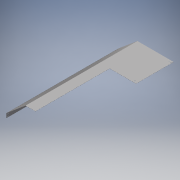
# Autodesk Inventor part: MC Part2
Saved by Autodesk Inventor 2016 (Build 200138000, 138)
## iProperties
Created: 2017-10-17
Part Number: MC Part2
Material: Steel, Mild
Document SubType Name: Sheet Metal
Designer: m207653
Density: 7.85 g/cm^3
Sheet Metal Rule: ms steel
Appearance: Semi-Polished
Flat Pattern Width: 99.3305 cm
Flat Pattern Length: 169.5 cm
Flat Pattern Area: 16836.5 cm^2
Sheet Metal Width: 993.305 mm
Sheet Metal Length: 1695.000 mm
Sheet Metal Area: 1683652.545 mm^2
Author: m207653
Autodesk Inventor part; units mm, degrees
ref_plane "YZ Plane" through (0, 0, 0) normal (1, 0, 0) x (0, 1, 0)
ref_plane "XZ Plane" through (0, 0, 0) normal (0, 1, 0) x (-1, 0, 0)
ref_plane "XY Plane" through (0, 0, 0) normal (0, 0, 1) x (1, 0, 0)
sketch "Sketch1" plane through (0, 0, 0) normal (0, 0, 1) x (1, 0, 0)
  line L0 (0, 0) -> (150, 0)
  line L1 (0, 0) -> (0, 1695)
  line L2 (0, 1695) -> (550, 1695)
  line L3 (550, 1695) -> (550, 1125)
  line L4 (550, 1125) -> (150, 1125)
  line L5 (150, 1125) -> (150, 0)
  dimension "d0" = 150
  dimension "d1" = 1695
  dimension "d2" = 550
  dimension "d3" = 570
  measures "d0" distance of L0.start L0.end
  measures "d1" distance of L0.start L1.end
  measures "d2" distance of L1.end L2.end
  measures "d3" distance of L2.end L3.end
extrude "Plate1" add sketch "Sketch1" along normal blind 1.6
sketch "Sketch2" plane through (1.0285, 0, 0.3743) normal (-0.6427876, 0, 0.7660444) x (0, -1, 0)
  line L0 (-1695, 0) -> (0, 0)
  line L1 (0, 0) -> (0, 380)
  line L2 (0, 380) -> (-1695, 380)
  line L3 (-1695, 380) -> (-1695, 0)
  constraints: 6 end point, 1 horizontal, 1 perpendicular, 1 vertical
edge flange "Flange1" height 380 angle 40 thickness 1.6 bend radius 1.6 thickness toward (-0.6427876, 0, 0.7660444) relief straight relief width 1.6 relief depth 0.8 edges at (0, 847.5, 1.6) wall of the first edge with corners at (1.0285, 1695, 0.3743) (1.0285, 0, 0.3743) (-290.0684, 0, -243.885) (-290.0684, 1695, -243.885)
bend "Bend1"
corner "Corner1"
sketch "Sketch4" plane through (-289.4969, 0, -242.6593) normal (-1, 0, 0) x (0, -1, 0)
  line L0 (-1695, 0) -> (0, 0)
  line L1 (0, 0) -> (0, 65)
  line L2 (0, 65) -> (-1695, 65)
  line L3 (-1695, 65) -> (-1695, 0)
  constraints: 6 end point, 1 horizontal, 1 perpendicular, 1 vertical
edge flange "Flange2" height 65 angle -50 thickness 1.6 bend radius 1.6 thickness toward (-1, 0, 0) relief straight relief width 1.6 relief depth 0.8 edges at (-291.0969, 847.5, -242.6593) wall of the first edge with corners at (-289.4969, 1695, -242.6593) (-289.4969, 0, -242.6593) (-289.4969, 0, -307.6593) (-289.4969, 1695, -307.6593)
bend "Bend2"
corner "Corner2"
sketch "Sketch6" plane through (-291.0969, 0, -307.6593) normal (-1, 0, 0) x (0, 0, 1)
  line L0 (0, 1695) -> (0, 0) projected
  line L1 (0, 0) -> (60, 0)
  line L2 (0, 0) -> (63.5078, 0) projected
  line L3 (60, 0) -> (60, 1695)
  line L4 (63.5078, 1695) -> (0, 1695) projected
  line L5 (60, 1695) -> (0, 1695)
  line L6 (0, 1695) -> (0, 0)
  circle A0 centre (45, 1670) radius 6
  circle A1 centre (15, 1670) radius 6
  circle A2 centre (45, 25) radius 6
  circle A3 centre (15, 25) radius 6
  point P0 (307.6593, 0)
  dimension "d39" = 60
  dimension "d40" = 12
  dimension "d41" = 12
  dimension "d42" = 25
  dimension "d43" = 25
  dimension "d44" = 15
  dimension "d45" = 15
  dimension "d46" = 12
  dimension "d47" = 12
  dimension "d48" = 25
  dimension "d49" = 25
  dimension "d77" = 15
  dimension "d78" = 15
  constraints: 8 end point, 4 centre point, 2 collinear, 2 point on line, 1 perpendicular
  measures "d39" distance of L0.end L1.end
  measures "d40" diameter of A0
  measures "d41" diameter of A1
  measures "d42" distance from line of L4 A0.centre
  measures "d43" distance from line of L4 A1.centre
  measures "d44" distance from line of L3 A0.centre
  measures "d45" distance from line of L0 A1.centre
  measures "d46" diameter of A2
  measures "d47" diameter of A3
  measures "d48" distance from line of L1 A2.centre
  measures "d49" distance from line of L1 A3.centre
  measures "d77" distance from line of L3 A2.centre
  measures "d78" distance from line of L0 A3.centre
hole "Hole2" at (-291.0969, 1670, -262.6593) at (-291.0969, 1670, -292.6593) at (-291.0969, 25, -262.6593) at (-291.0969, 25, -292.6593) direction (1, 0, 0) diameter 12 end through all
sketch "Sketch7" plane through (0, 0, 1.6) normal (0, 0, 1) x (1, 0, 0)
  line L0 (1.1647, 1695) -> (550, 1695) projected
  line L1 (490, 1695) -> (490, 1125)
  line L2 (550, 1125) -> (150, 1125) projected
  line L3 (550, 1695) -> (550, 1125) projected
  circle A0 centre (535, 1670) radius 6
  circle A1 centre (505, 1670) radius 6
  circle A2 centre (535, 1150) radius 6
  circle A3 centre (505, 1150) radius 6
  point P0 (0, 0)
  dimension "d57" = 60
  dimension "d58" = 12
  dimension "d59" = 12
  dimension "d60" = 15
  dimension "d61" = 15
  dimension "d62" = 25
  dimension "d63" = 25
  dimension "d64" = 12
  dimension "d65" = 12
  dimension "d66" = 25
  dimension "d67" = 25
  dimension "d75" = 15
  dimension "d76" = 15
  constraints: 4 centre point, 2 end point, 2 point on line, 1 vertical
  measures "d57" distance between parallel lines of L1 L3
  measures "d58" diameter of A0
  measures "d59" diameter of A1
  measures "d60" distance from line of L3 A0.centre
  measures "d61" distance from line of L1 A1.centre
  measures "d62" distance from line of L0 A0.centre
  measures "d63" distance from line of L0 A1.centre
  measures "d64" diameter of A2
  measures "d65" diameter of A3
  measures "d66" distance from line of L2 A2.centre
  measures "d67" distance from line of L2 A3.centre
  measures "d75" distance from line of L1 A3.centre
  measures "d76" distance from line of A2.centre L3
hole "Hole3" at (535, 1670, 1.6) at (505, 1670, 1.6) at (535, 1150, 1.6) at (505, 1150, 1.6) direction (0, 0, -1) diameter 12 end through all
equation "\"d55\" = Thickness"
equation "\"d73\" = Thickness"
equation "\"d5\" = BendReliefWidth"
equation "\"d6\" = BendReliefDepth"
equation "\"d7\" = MinimumRemnant"
equation "\"d8\" = BendRadius"
equation "\"d11\" = BendRadius"
equation "\"d12\" = CornerReliefSize"
equation "\"d13\" = GapSize"
equation "\"d14\" = JacobiRadiusSize"
equation "\"d28\" = BendReliefWidth"
equation "\"d29\" = BendReliefDepth"
equation "\"d30\" = MinimumRemnant"
equation "\"d31\" = BendRadius"
equation "\"d34\" = BendRadius"
equation "\"d35\" = CornerReliefSize"
equation "\"d36\" = GapSize"
equation "\"d37\" = JacobiRadiusSize"
equation "\"BendRadius\" = Thickness"
equation "\"BendReliefWidth\" = Thickness"
equation "\"BendReliefDepth\" = 0.5 * Thickness"
equation "\"CornerReliefSize\" = 4 * Thickness"
equation "\"MinimumRemnant\" = 2 * Thickness"
equation "\"TransitionRadius\" = BendRadius"
equation "\"JacobiRadiusSize\" = BendRadius"
equation "\"GapSize\" = Thickness"
equation "\"d4\" = BendRadius"
equation "\"Thickness\" = 1.6"
body "Solid1"
